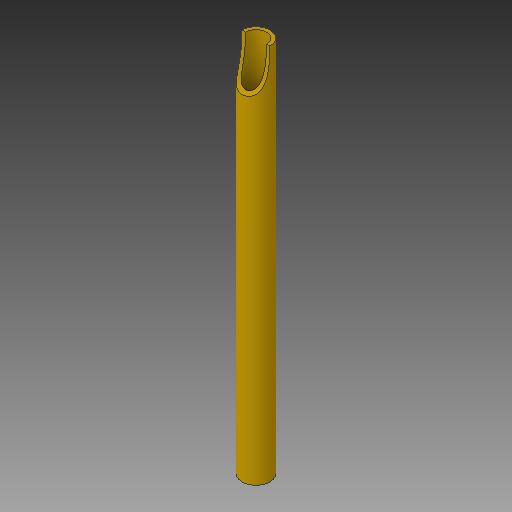
# Autodesk Inventor part: pin
Saved by Autodesk Inventor 2018 (Build 220112000, 112)
## iProperties
Created: 2019-04-17
Part Number: pin
Material: Generic
Document SubType Name: Modeling
Designer: ZEUSLAP
Density: 1 g/cm^3
Appearance: Default
Mass: 0.0354189 g
Surface Area: 2.8738 cm^2
Volume: 0.0354189 cm^3
Author: ZEUSLAP
Autodesk Inventor part; units mm, degrees
ref_plane "YZ Plane" through (0, 0, 0) normal (1, 0, 0) x (0, 1, 0)
ref_plane "XZ Plane" through (0, 0, 0) normal (0, 1, 0) x (-1, 0, 0)
ref_plane "XY Plane" through (0, 0, 0) normal (0, 0, 1) x (1, 0, 0)
sketch "Sketch1" plane through (0, 0, 0) normal (0, 1, 0) x (-1, 0, 0)
  circle A0 centre (0, 0) radius 1
  circle A1 centre (0, 0) radius 0.75
  dimension "d0" = 2
  dimension "d1" = 1.5
  constraints: 2 centre point, 2 coincident
  measures "d0" diameter of A0
  measures "d1" diameter of A1
extrude "Extrusion1" add sketch "Sketch1" along normal blind 27
sketch "Sketch2" plane through (0, 0, 0) normal (1, 0, 0) x (0, 1, 0)
  line L0 (0, 1) -> (27, 1) construction
  line L1 (27, 0) -> (24.5005, 0) construction
  line L2 (27, 0) -> (24.5005, 0) construction
  line L3 (24.5005, 0) -> (24, 1) construction
  spline S0 degree 2 poles (27, 0) (24.5005, 0) (24, 1) knots 1 1 1 2 2 2
  line L4 (24, 1) -> (27.2057, 2.7706)
  line L5 (27.2057, 2.7706) -> (28.0027, -0.4432)
  line L6 (28.0027, -0.4432) -> (27, 0)
  point P0 (0, 0)
  constraints: 8 end point, 1 coincident, 1 collinear, 1 horizontal, 1 point on line, 3 other
extrude "Extrusion2" cut sketch "Sketch2" against normal blind 1 and the other way blind 1
body "Solid1"
